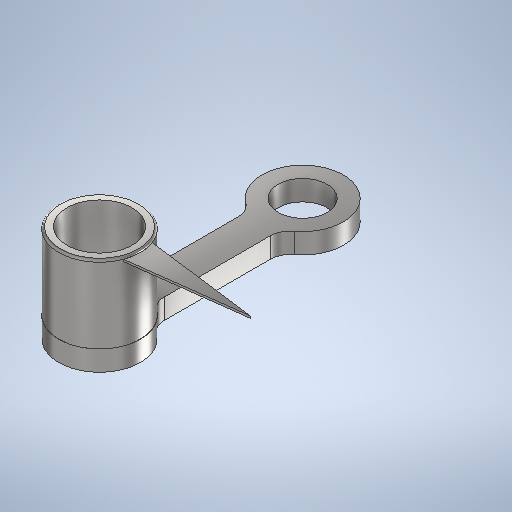
# Autodesk Inventor part: 203 part 1
Saved by Autodesk Inventor 2025.1 (Build 291241000, 241)
## iProperties
Created: 2024-09-02
Part Number: 203 part 1
Material: Steel, Alloy
Document SubType Name: Modeling
Designer: ffogue
Density: 7.73 g/cm^3
Appearance: Semi-Polished
Author: ffogue
Autodesk Inventor part; units mm, degrees
ref_plane "YZ Plane" through (0, 0, 0) normal (1, 0, 0) x (0, 1, 0)
ref_plane "XZ Plane" through (0, 0, 0) normal (0, 1, 0) x (-1, 0, 0)
sketch "Sketch1" plane through (0, 0, 0) normal (0, 0, 1) x (1, 0, 0)
  line L0 (-4, 15.8348) -> (-4, -15.8348)
  line L1 (4, 15.8348) -> (4, -15.8348)
  arc A0 (4, 15.8348) -> (-4, 15.8348) centre (0, 25) ccw
  arc A1 (-4, -15.8348) -> (4, -15.8348) centre (0, -25) ccw
  circle A2 centre (0, 25) radius 6
  circle A3 centre (0, -25) radius 4
  point P0 (0, 0)
  point P1 (-4, 0)
  dimension "d0" = 50
  dimension "d1" = 8
  dimension "d2" = 4
  dimension "d3" = 10
  dimension "d4" = 10
  dimension "d5" = 12
  dimension "d6" = 8
  constraints: 4 centre point, 4 end point, 4 point on circle, 3 horizontal alignment, 2 coincident, 2 vertical, 1 midpoint
  measures "d0" distance of A1.centre A0.centre
  measures "d1" distance between parallel lines of L1 L0
  measures "d2" distance of point (-4, 0) point (0, 0)
  measures "d3" radius of A0
  measures "d4" radius of A1
  measures "d5" diameter of A2
  measures "d6" diameter of A3
extrude "Extrusion1" add sketch "Sketch1" against normal blind 5
fillet "Fillet1" radius 5 4 edges at (4, 15.8348, -2.5) (-4, 15.8348, -2.5) (4, -15.8348, -2.5) (-4, -15.8348, -2.5)
sketch "Sketch2" plane through (0, 0, 0) normal (0, 0, 1) x (1, 0, 0)
  circle A0 centre (0, -25) radius 4 projected
  circle A1 centre (0, -25) radius 10.0559
  point P0 (0, 0)
  constraints: 1 centre point, 1 coincident
extrude "Extrusion2" add sketch "Sketch2" along normal blind 19
sketch "Sketch3" plane through (0, -25, 19) normal (0, 0, 1) x (1, 0, 0)
  circle A0 centre (0, 0) radius 10.0559 projected
  point P0 (0, 25)
  constraints: 1 coincident
hole "Hole1" at (0, -25, 19) direction (0, 0, -1) diameter 16 depth 12.5
fillet "Fillet2" radius 0.5 1 edges at (-10.0559, -25, 19)
ref_plane "Work Plane1" through (0, 0, 18) normal (0, 0, 1) x (1, 0, 0)
sketch "Sketch5" plane through (0, 0, 18) normal (0, 0, 1) x (1, 0, 0)
  arc A0 (-6, -17) -> (6, -17) centre (0, -25) ccw projected
  line L0 (9.3495, -21.4523) -> (37.147, -25)
  line L1 (37.147, -25) -> (9.3495, -28.5477)
  line L2 (0, -25) -> (37.147, -25) construction
  arc A1 (9.3495, -28.5477) -> (9.3495, -21.4523) centre (0.7935, -25) ccw
  point P0 (0, 0)
  constraints: 6 end point, 4 point on circle, 1 centre point, 1 horizontal, 1 symmetric about line
extrude "Extrusion3" add sketch "Sketch5" along normal blind 0.5 separate body contours A1 L0 L1
body "Solid1"
